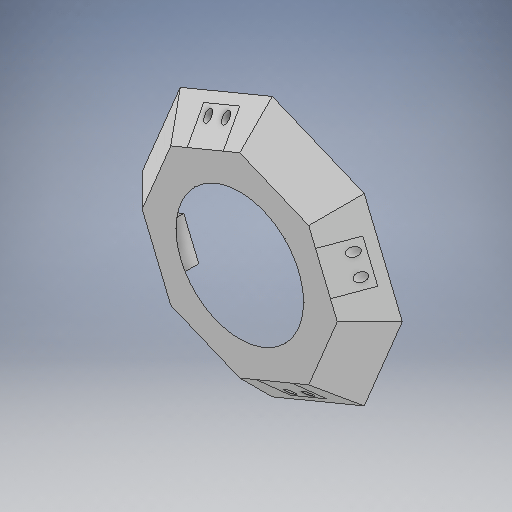
# Autodesk Inventor part: Base_Chanf
Saved by Autodesk Inventor 2025.2 (Build 292293000, 293)
## iProperties
Created: 2025-04-01
Part Number: Base_Chanf
Material: Generic
Document SubType Name: Modeling
Designer: Tiago
Density: 1 g/cm^3
Appearance: Default
Author: Tiago
Autodesk Inventor part; units mm, degrees
ref_plane "YZ Plane" through (0, 0, 0) normal (1, 0, 0) x (0, 1, 0)
ref_plane "XZ Plane" through (0, 0, 0) normal (0, 1, 0) x (-1, 0, 0)
sketch "Sketch1" plane through (0, 0, 0) normal (0, 0, 1) x (1, 0, 0)
  circle A0 centre (0, 0) radius 100
  line L0 (0, 100) -> (70.7107, 70.7107)
  line L1 (70.7107, 70.7107) -> (100, 0)
  line L2 (100, 0) -> (70.7107, -70.7107)
  line L3 (70.7107, -70.7107) -> (0, -100)
  line L4 (0, -100) -> (-70.7107, -70.7107)
  line L5 (-70.7107, -70.7107) -> (-100, 0)
  line L6 (-100, 0) -> (-70.7107, 70.7107)
  line L7 (-70.7107, 70.7107) -> (0, 100)
  line L8 (66.8838, 66.8838) -> (0, 94.588)
  line L9 (0, 94.588) -> (-66.8838, 66.8838)
  line L10 (-66.8838, 66.8838) -> (-94.588, 0)
  line L11 (-94.588, 0) -> (-66.8838, -66.8838)
  line L12 (-66.8838, -66.8838) -> (0, -94.588)
  line L13 (0, -94.588) -> (66.8838, -66.8838)
  line L14 (66.8838, -66.8838) -> (94.588, 0)
  line L15 (94.588, 0) -> (66.8838, 66.8838)
  line L16 (80.7359, 33.4419) -> (62.2584, 25.7883) construction
  line L17 (86.4762, 19.5837) -> (67.9986, 11.9301)
  line L18 (74.9957, 47.3001) -> (56.5181, 39.6464)
  line L19 (80.7359, 33.4419) -> (62.2584, 25.7883) construction
  line L20 (62.2584, 25.7883) -> (56.5181, 39.6464)
  line L21 (62.2584, 25.7883) -> (67.9986, 11.9301)
  line L22 (74.9957, 47.3001) -> (86.4762, 19.5837)
  line L23 (-19.5837, 86.4762) -> (-11.9301, 67.9986)
  line L24 (-25.7883, 62.2584) -> (-11.9301, 67.9986)
  line L25 (-25.7883, 62.2584) -> (-39.6464, 56.5181)
  line L26 (-47.3001, 74.9957) -> (-39.6464, 56.5181)
  line L27 (-47.3001, 74.9957) -> (-19.5837, 86.4762)
  line L28 (-86.4762, -19.5837) -> (-67.9986, -11.9301)
  line L29 (-62.2584, -25.7883) -> (-67.9986, -11.9301)
  line L30 (-62.2584, -25.7883) -> (-56.5181, -39.6464)
  line L31 (-74.9957, -47.3001) -> (-56.5181, -39.6464)
  line L32 (-74.9957, -47.3001) -> (-86.4762, -19.5837)
  line L33 (19.5837, -86.4762) -> (11.9301, -67.9986)
  line L34 (25.7883, -62.2584) -> (11.9301, -67.9986)
  line L35 (25.7883, -62.2584) -> (39.6464, -56.5181)
  line L36 (47.3001, -74.9957) -> (39.6464, -56.5181)
  line L37 (47.3001, -74.9957) -> (19.5837, -86.4762)
  circle A1 centre (78.9867, 24.5994) radius 3
  circle A2 centre (73.2464, 38.4576) radius 3
  line L38 (83.6061, 26.5128) -> (76.677, 23.6427) construction
  line L39 (77.8658, 40.371) -> (70.9367, 37.5009) construction
  circle A3 centre (-24.5994, 78.9867) radius 3
  circle A4 centre (-38.4576, 73.2464) radius 3
  circle A5 centre (-78.9867, -24.5994) radius 3
  circle A6 centre (-73.2464, -38.4576) radius 3
  circle A7 centre (24.5994, -78.9867) radius 3
  circle A8 centre (38.4576, -73.2464) radius 3
  dimension "d0" = 200
  dimension "d22" = 5
  dimension "d23" = 15
  dimension "d24" = 15
  dimension "d25" = 20
  dimension "d28" = 360
  dimension "d46" = 6
  dimension "d47" = 6
  dimension "d54" = 7.5
  dimension "d55" = 7.5
  dimension "d58" = 360
  constraints: 80 end point, 8 centre point, 6 point on line, 3 perpendicular, 2 coincident, 2 parallel, 1 collinear, 1 midpoint, 1 vertical alignment, 84 other
  measures "d22" distance between parallel lines of L0 L8
  measures "d23" distance between parallel lines of L16 L17
  measures "d24" distance between parallel lines of L16 L18
  measures "d25" distance of L16.end L16.start
  measures "d46" diameter of A1
  measures "d47" diameter of A2
  measures "d54" distance of L38.start L38.end
  measures "d55" distance of L39.start L39.end
ref_plane "Work Plane1" through (0, 0, 25) normal (0, 0, 1) x (1, 0, 0)
sketch "Sketch2" plane through (0, 0, 25) normal (0, 0, 1) x (1, 0, 0)
  circle A0 centre (0, 0) radius 75
  line L0 (0, 75) -> (53.033, 53.033)
  line L1 (53.033, 53.033) -> (75, 0)
  line L2 (75, 0) -> (53.033, -53.033)
  line L3 (53.033, -53.033) -> (0, -75)
  line L4 (0, -75) -> (-53.033, -53.033)
  line L5 (-53.033, -53.033) -> (-75, 0)
  line L6 (-75, 0) -> (-53.033, 53.033)
  line L7 (-53.033, 53.033) -> (0, 75)
  circle A1 centre (0, 0) radius 49
  dimension "d3" = 150
  dimension "d4" = 98
  constraints: 16 end point, 3 coincident, 1 centre point, 1 vertical alignment, 19 other
  measures "d4" diameter of A1
loft "Loft3" add profiles "Sketch1", "Sketch2" contours L2 L3 L4 L5 L6 L7 L0 L1 | L15 L18 L20 L21 L17 L14 L13 L36 L35 L34 L33 L12 L11 L31 L30 L29 L28 L10 L9 L26 L25 L24 L23 L8 | L15 L17 L21 L20 L18 | L23 L24 L25 L26 L9 | L13 L33 L34 L35 L36 | L28 L29 L30 L31 L11 | A1 | A2 | A3 | A4 | A5 | A6 | A7 | A8 / L2 L3 L4 L5 L6 L7 L0 L1 | A1
loft "Loft4" cut profiles "Sketch1", "Sketch2" contours L15 L18 L20 L21 L17 L14 L13 L36 L35 L34 L33 L12 L11 L31 L30 L29 L28 L10 L9 L26 L25 L24 L23 L8 | L15 L17 L21 L20 L18 | L23 L24 L25 L26 L9 | L13 L33 L34 L35 L36 | L28 L29 L30 L31 L11 | A1 | A2 | A3 | A4 | A5 | A6 | A7 | A8 / A1
extrude "Extrusion2" add sketch "Sketch1" along normal blind 25 contours L15 L17 L21 L20 L18 | L23 L24 L25 L26 L9 | L13 L33 L34 L35 L36 | L28 L29 L30 L31 L11 | A1 | A2 | A3 | A4 | A5 | A6 | A7 | A8
ref_plane "Work Plane3" through (-13.8582, -5.7403, 12.6568) normal (-0.3826834, 0.9238795, 0) x (0.9238795, 0.3826834, 0)
ref_plane "Work Plane4" through (-5.7403, 13.8582, 12.6568) normal (0.9238795, 0.3826834, 0) x (0, 0, -1)
sketch "Sketch4" plane through (-5.7403, 13.8582, 12.6568) normal (0.9238795, 0.3826834, 0) x (0, 0, -1)
  line L0 (12.6568, 52.388) -> (-0.3682, 52.388) projected
  line L1 (-12.3432, 34) -> (-12.3432, 72.388) projected
  line L2 (-12.3432, 72.388) -> (7.2448, 72.388) projected
  line L3 (7.2448, 72.388) -> (12.6568, 77.388) projected
  line L4 (12.6568, 77.388) -> (12.6568, 52.388) projected
  line L5 (-0.3682, -82.388) -> (12.6568, -82.388) projected
  line L6 (12.6568, -82.388) -> (12.6568, -107.388) projected
  line L7 (12.6568, -107.388) -> (7.2448, -102.388) projected
  line L8 (7.2448, -102.388) -> (-12.3432, -102.388) projected
  line L9 (-12.3432, -102.388) -> (-12.3432, -64) projected
  line L10 (-12.3432, -84.291) -> (7.2448, -102.388)
  line L11 (7.2448, -102.388) -> (-12.3432, -102.388) projected
  line L12 (7.2448, -102.388) -> (-12.3432, -102.388)
  line L13 (-12.3432, -102.388) -> (-12.3432, -84.291)
  line L14 (12.6568, 77.388) -> (-12.3432, 54.291) projected
  line L15 (-12.3432, 54.291) -> (-12.3432, 72.388)
  line L16 (-12.3432, 72.388) -> (7.2448, 72.388)
  line L17 (7.2448, 72.388) -> (-12.3432, 54.291)
  point P0 (12.6568, -15)
  constraints: 12 end point, 5 collinear, 2 point on line, 2 other
sketch "Sketch5" plane through (-13.8582, -5.7403, 12.6568) normal (-0.3826834, 0.9238795, 0) x (0.9238795, 0.3826834, 0)
  line L0 (-52.388, 12.6568) -> (-52.388, -0.3682) projected
  line L1 (-34, -12.3432) -> (-72.388, -12.3432) projected
  line L2 (-72.388, -12.3432) -> (-72.388, 7.2448) projected
  line L3 (-72.388, 7.2448) -> (-77.388, 12.6568) projected
  line L4 (-77.388, 12.6568) -> (-52.388, 12.6568) projected
  line L5 (82.388, -0.3682) -> (82.388, 12.6568) projected
  line L6 (82.388, 12.6568) -> (107.388, 12.6568) projected
  line L7 (107.388, 12.6568) -> (102.388, 7.2448) projected
  line L8 (102.388, 7.2448) -> (102.388, -12.3432) projected
  line L9 (102.388, -12.3432) -> (64, -12.3432) projected
  line L10 (84.291, -12.3432) -> (102.388, 7.2448)
  line L11 (102.388, 7.2448) -> (102.388, -12.3432)
  line L12 (102.388, -12.3432) -> (84.291, -12.3432)
  line L13 (-72.388, 7.2448) -> (-72.388, -12.3432)
  line L14 (-72.388, -12.3432) -> (-40.903, -12.3432)
  line L15 (-72.388, 7.2448) -> (-54.291, -12.3432)
  point P0 (15, 12.6568)
  constraints: 12 end point, 4 collinear, 3 point on line, 2 other
extrude "Extrusion4" cut sketch "Sketch5" along normal mid plane 30
extrude "Extrusion5" cut sketch "Sketch4" along normal mid plane 30
extrude "Extrusion6" cut sketch "Sketch1" along normal blind 25 contours A1 | A2 | A3 | A4 | A5 | A6 | A7 | A8
body "Solid2"
